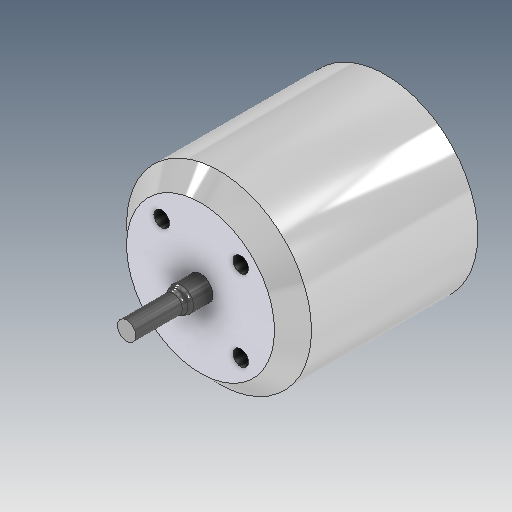
# Autodesk Inventor part: DCMotorv2
Saved by Autodesk Inventor 2021 (Build 250183000, 183)
## iProperties
Created: 2021-06-25
Part Number: DCMotorv2
Material: Generic
Document SubType Name: Modeling
Designer: RahulRC
Density: 1 g/cm^3
Appearance: Default
Author: RahulRC
Autodesk Inventor part; units mm, degrees
ref_plane "YZ Plane" through (0, 0, 0) normal (1, 0, 0) x (0, 1, 0)
ref_plane "XZ Plane" through (0, 0, 0) normal (0, 1, 0) x (-1, 0, 0)
ref_plane "XY Plane" through (0, 0, 0) normal (0, 0, 1) x (1, 0, 0)
sketch "Sketch1" plane through (0, 0, 0) normal (0, 0, 1) x (1, 0, 0)
  circle A0 centre (0, 0) radius 15
  constraints: 1 centre point, 1 coincident
extrude "Extrusion1" add sketch "Sketch1" along normal blind 30
chamfer "Chamfer1" distance 3 angle 45 1 edges at (-15, 0, 30)
sketch "Sketch2" plane through (0, 0, 30) normal (0, 0, 1) x (1, 0, 0)
  circle A0 centre (0, 0) radius 2
  constraints: 1 centre point, 1 coincident
extrude "Extrusion2" add sketch "Sketch2" along normal blind 4
sketch "Sketch3" plane through (0, 0, 34) normal (0, 0, 1) x (1, 0, 0)
  circle A0 centre (0, 0) radius 1.5
  constraints: 1 centre point
extrude "Extrusion3" add sketch "Sketch3" along normal blind 8
fillet "Fillet1" radius 1 2 edges at (-2, 0, 34) (-1.5, 0, 34)
sketch "Sketch4" plane through (0, 0, 30) normal (0, 0, 1) x (1, 0, 0)
  point P0 (0, 0)
sketch "Sketch5" plane through (0, 0, 30) normal (0, 0, 1) x (1, 0, 0)
  circle A0 centre (0, 0) radius 12 projected
  circle A1 centre (6.5184, -6.551) radius 1.25
  circle A2 centre (-6.3094, 6.5625) radius 1.25
  circle A3 centre (6.5184, 6.5625) radius 1.25
  circle A4 centre (-6.4741, -6.551) radius 1.25
  constraints: 4 centre point
extrude "Extrusion4" cut sketch "Sketch5" against normal blind 8 contours A1 | A2 | A3 | A4
sketch "Sketch6" plane through (0, 0, 0) normal (0, 0, -1) x (-1, 0, 0)
  point P0 (0, 0)
hole "Hole1" at (0, 0, 0) direction (0, 0, 1) diameter 4 depth 10 tip angle 120
body "Solid1"
